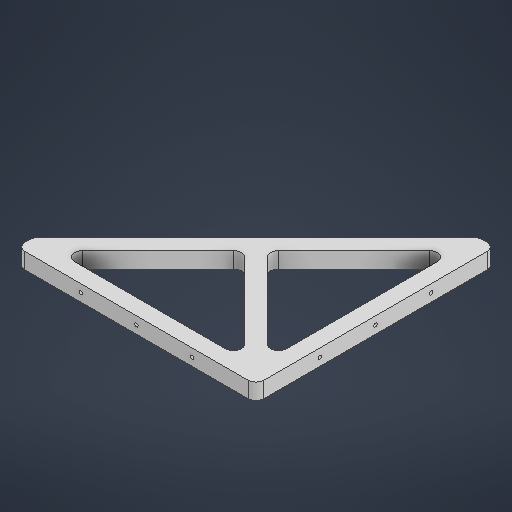
# Autodesk Inventor part: Aufhängung_Gerüst
Saved by Autodesk Inventor 2027 (Build 310192060, 192F)
## iProperties
Created: 2026-07-21
Part Number: Aufhängung_Gerüst
Material: Generic
Document SubType Name: Modeling
Designer: kw
Density: 1 g/cm^3
Appearance: Default
Author: kw
Autodesk Inventor part; units mm, degrees
ref_plane "YZ Plane" through (0, 0, 0) normal (1, 0, 0) x (0, 1, 0)
ref_plane "XZ Plane" through (0, 0, 0) normal (0, 1, 0) x (-1, 0, 0)
ref_plane "XY Plane" through (0, 0, 0) normal (0, 0, 1) x (1, 0, 0)
sketch "Sketch1" plane through (0, 0, 0) normal (0, 1, 0) x (-1, 0, 0)
  line L0 (0, 0) -> (20, 0)
  line L1 (20, 0) -> (20, -300)
  line L2 (20, -300) -> (0, -300)
  line L3 (0, -300) -> (0, 0)
  line L4 (0, 0) -> (300, 0)
  line L5 (300, 0) -> (300, -20)
  line L6 (300, -20) -> (0, -20)
  line L7 (0, -20) -> (0, 0)
  line L8 (300, -20) -> (20, -300)
  line L9 (285.8579, -5.8579) -> (5.8579, -285.8579)
  line L10 (-7.0711, -7.0711) -> (152.9289, -167.0711)
  line L11 (7.0711, 7.0711) -> (167.0711, -152.9289)
  point P0 (138.7868, -152.9289)
  point P1 (20, -271.7157)
  point P2 (20, -34.1421)
  point P3 (152.9289, -138.7868)
  point P4 (34.1421, -20)
  point P5 (271.7157, -20)
  dimension "d32" = 20
  dimension "d33" = 300
  dimension "d34" = 300
  dimension "d35" = 20
  dimension "d36" = 20
  constraints: 24 end point, 5 parallel, 2 horizontal, 2 perpendicular
  measures "d32" distance of L1.end L2.end
  measures "d33" distance of L0.end L1.end
  measures "d34" distance of L5.end L6.end
  measures "d35" distance of L4.end L5.end
  measures "d36" distance between parallel lines of L8 L9
extrude "Extrusion1" add sketch "Sketch1" along normal blind 20 contours L0 L11 L1 L6 L10 L3 | L0 L1 L11 | L10 L6 L3 | L4 L5 L6 L11 L1 | L11 L6 L1 | L6 L10 L1 L2 L3 | L6 L1 L10 | L6 L11 L9 L10 L1 | L8 L11 L9 L6 | L11 L8 L10 L9 | L1 L9 L10 L8
fillet "Fillet1" radius 10 11 edges at (-300, 10, 0) (-300, 10, -20) (-271.7157, 10, -20) (-152.9289, 10, -138.7868) (-138.7868, 10, -152.9289) (-34.1421, 10, -20) (-20, 10, -34.1421) (0, 10, 0) (-20, 10, -300) (0, 10, -300) (-20, 10, -271.7157)
sketch "Sketch3" plane through (-290, 0, 0) normal (0, 0, 1) x (1, 0, 0)
  line L0 (0, 0) -> (0, 20) projected
  line L1 (0, 10) -> (70, 10)
  line L2 (70, 10) -> (140, 10)
  line L3 (140, 10) -> (210, 10)
  line L4 (210, 10) -> (280, 10)
  point P0 (290, 0)
  dimension "d39" = 70
  dimension "d40" = 70
  dimension "d41" = 70
  dimension "d42" = 70
  constraints: 8 end point, 3 point on line, 1 horizontal, 1 midpoint
  measures "d39" distance of L1.start L1.end
  measures "d40" distance of L1.end L2.end
  measures "d41" distance of L2.end L3.end
  measures "d42" distance of L3.end L4.end
hole "Hole2" at (-220, 10, 0) at (-150, 10, 0) at (-80, 10, 0) direction (0, 0, -1) diameter 4.3 depth 20 clearance for "Socket Head Cap Screw ISO 4762" size "M4" standard "ISO"
sketch "Sketch4" plane through (0, 0, -10) normal (1, 0, 0) x (0, 0, -1)
  line L0 (280, 20) -> (280, 0) projected
  line L1 (280, 10) -> (210, 10)
  line L2 (210, 10) -> (140, 10)
  line L3 (140, 10) -> (70, 10)
  line L4 (70, 10) -> (0, 10)
  point P0 (-10, 0)
  dimension "d50" = 70
  dimension "d51" = 70
  dimension "d52" = 70
  dimension "d53" = 70
  constraints: 8 end point, 3 point on line, 1 horizontal, 1 midpoint
  measures "d50" distance of L1.start L1.end
  measures "d51" distance of L1.end L2.end
  measures "d52" distance of L2.end L3.end
  measures "d53" distance of L3.end L4.end
hole "Hole3" at (0, 10, -220) at (0, 10, -150) at (0, 10, -80) direction (-1, 0, 0) diameter 4.3 depth 20 clearance for "Socket Head Cap Screw ISO 4762" size "M4" standard "ISO"
body "Solid1"
